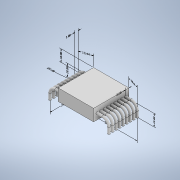
# Autodesk Inventor part: Деталь2
Saved by Autodesk Inventor 2021 (Build 250183000, 183)
## iProperties
Created: 2022-10-18
Part Number: Деталь2
Material: Типовые
Document SubType Name: Modeling
Designer: 22-91-12
Density: 1 g/cm^3
Appearance: По умолчанию
Author: 22-91-12
Autodesk Inventor part; units mm, degrees
ref_plane "YZ Plane" through (0, 0, 0) normal (1, 0, 0) x (0, 1, 0)
ref_plane "XZ Plane" through (0, 0, 0) normal (0, 1, 0) x (-1, 0, 0)
ref_plane "XY Plane" through (0, 0, 0) normal (0, 0, 1) x (1, 0, 0)
sketch "Эскиз1" plane through (0, 0, 0) normal (0, 1, 0) x (-1, 0, 0)
  line L0 (6.5605, 11.4911) -> (-23.4395, 11.4911)
  line L1 (-23.4395, 11.4911) -> (-23.4395, -18.5089)
  line L2 (-23.4395, -18.5089) -> (6.5605, -18.5089)
  line L3 (6.5605, -18.5089) -> (6.5605, 11.4911)
  point P0 (0, 0)
  dimension "d0" = 30
  dimension "d1" = 30
  constraints: 8 end point, 2 parallel, 1 horizontal, 1 perpendicular
  measures "d0" distance of L2.end L1.end
  measures "d1" distance of L1.end L0.end
extrude "Выдавливание1" add sketch "Эскиз1" along normal blind 10
sketch "Эскиз2" plane through (23.4395, 0, 11.4911) normal (1, 0, 0) x (0, 0, -1)
  line L0 (0, 0) -> (0, 10) projected
  circle A0 centre (3, 5) radius 1
  circle A1 centre (6, 5) radius 1
  circle A2 centre (9, 5) radius 1
  circle A3 centre (12, 5) radius 1
  circle A4 centre (15, 5) radius 1
  circle A5 centre (18, 5) radius 1
  circle A6 centre (21, 5) radius 1
  circle A7 centre (24, 5) radius 1
  circle A8 centre (27, 5) radius 1
  point P0 (11.4911, 0)
  constraints: 9 centre point
sketch3d "3D эскиз1"
  line L0 (23.4395, 5, 8.4911) -> (28.4395, 5, 8.4911)
  arc A0 (28.4395, 5, 8.4911) -> (33.4395, 0, 8.4911) centre (28.4395, 0, 8.4911) ccw
  line L1 (33.4395, 0, 8.4911) -> (33.4395, -5, 8.4911)
  dimension "d24" = 10
  dimension "d25" = 10
  dimension "d26" = 10
  dimension "d27" = 10
  dimension "d28" = 10
  dimension "d29" = 10
  dimension "d30" = 10
  dimension "d31" = 10
  dimension "d32" = 10
  dimension "d33" = 10
  dimension "d34" = 10
  dimension "d35" = 10
  dimension "d36" = 10
  dimension "d37" = 10
  dimension "d38" = 10
  dimension "d39" = 10
  dimension "d40" = 10
  dimension "d41" = 10
  dimension "d42" = 5
  dimension "d43" = 5
  dimension "d44" = 5
  dimension "d45" = 5
  dimension "d46" = 5
  dimension "d47" = 5
sweep "Сдвиг1" add profiles "Эскиз2" path "3D эскиз1"
sketch "Эскиз3" plane through (-6.5605, 0, -18.5089) normal (-1, 0, 0) x (0, 0, 1)
  line L0 (0, 0) -> (0, 10) projected
  circle A0 centre (3, 5) radius 1 projected
  line L1 (0, 5) -> (3, 5)
  circle A1 centre (6, 5) radius 1 projected
  line L2 (3, 5) -> (6, 5)
  circle A2 centre (9, 5) radius 1 projected
  line L3 (6, 5) -> (9, 5)
  circle A3 centre (12, 5) radius 1 projected
  line L4 (9, 5) -> (12, 5)
  circle A4 centre (15, 5) radius 1 projected
  line L5 (12, 5) -> (15, 5)
  circle A5 centre (18, 5) radius 1 projected
  line L6 (15, 5) -> (18, 5)
  circle A6 centre (21, 5) radius 1 projected
  line L7 (18, 5) -> (21, 5)
  circle A7 centre (24, 5) radius 1 projected
  line L8 (21, 5) -> (24, 5)
  circle A8 centre (27, 5) radius 1 projected
  line L9 (24, 5) -> (27, 5)
  line L10 (27, 5) -> (30, 5)
  circle A9 centre (3, 5) radius 1
  circle A10 centre (6, 5) radius 1
  circle A11 centre (9, 5) radius 1
  circle A12 centre (12, 5) radius 1
  circle A13 centre (15, 5) radius 1
  circle A14 centre (18, 5) radius 1
  circle A15 centre (21, 5) radius 1
  circle A16 centre (24, 5) radius 1
  circle A17 centre (27, 5) radius 1
  point P0 (18.5089, 0)
  dimension "d44" = 5
  dimension "d53" = 3
  dimension "d54" = 3
  dimension "d55" = 3
  dimension "d56" = 3
  dimension "d57" = 3
  dimension "d58" = 3
  dimension "d59" = 3
  dimension "d60" = 3
  dimension "d61" = 3
  dimension "d62" = 3
  dimension "d63" = 2
  dimension "d64" = 2
  dimension "d65" = 2
  dimension "d66" = 2
  dimension "d67" = 2
  dimension "d68" = 2
  dimension "d69" = 2
  dimension "d70" = 2
  dimension "d71" = 2
  constraints: 20 end point, 9 centre point, 9 coincident, 8 collinear, 1 horizontal, 1 midpoint, 1 point on line
  measures "d53" distance of L1.start L1.end
  measures "d54" distance of L1.end L2.end
  measures "d55" distance of L2.end L3.end
  measures "d56" distance of L3.end L4.end
  measures "d57" distance of L4.end L5.end
  measures "d58" distance of L5.end L6.end
  measures "d59" distance of L6.end L7.end
  measures "d60" distance of L7.end L8.end
  measures "d61" distance of L8.end L9.end
  measures "d62" distance of L9.end L10.end
  measures "d63" diameter of A9
  measures "d64" diameter of A10
  measures "d65" diameter of A11
  measures "d66" diameter of A12
  measures "d67" diameter of A13
  measures "d68" diameter of A14
  measures "d69" diameter of A15
  measures "d70" diameter of A16
  measures "d71" diameter of A17
sketch3d "3D эскиз2"
  line L0 (-6.5605, 5, -15.5089) -> (-11.5605, 5, -15.5089)
  arc A0 (-11.5605, 5, -15.5089) -> (-16.5605, 0, -15.5089) centre (-11.5605, 0, -15.5089) ccw
  line L1 (-16.5605, 0, -15.5089) -> (-16.5605, -5, -15.5089)
  dimension "d72" = 10
  dimension "d73" = 10
  dimension "d74" = 10
  dimension "d75" = 10
  dimension "d76" = 10
  dimension "d77" = 10
  dimension "d78" = 10
  dimension "d79" = 10
  dimension "d80" = 10
  dimension "d81" = 10
  dimension "d82" = 10
  dimension "d83" = 10
  dimension "d84" = 10
  dimension "d85" = 10
  dimension "d86" = 10
  dimension "d87" = 10
  dimension "d88" = 10
  dimension "d89" = 10
  dimension "d90" = 5
  dimension "d91" = 5
  dimension "d92" = 5
  dimension "d93" = 5
  dimension "d94" = 5
  dimension "d95" = 5
sweep "Сдвиг2" add profiles "Эскиз3" path "3D эскиз2"
equation "\"d43\" = d42"
equation "\"d44\" = d42"
equation "\"d45\" = d42"
equation "\"d46\" = d42"
equation "\"d47\" = d42"
equation "\"d91\" = d90"
equation "\"d92\" = d90"
equation "\"d93\" = d90"
equation "\"d94\" = d90"
equation "\"d95\" = d90"
